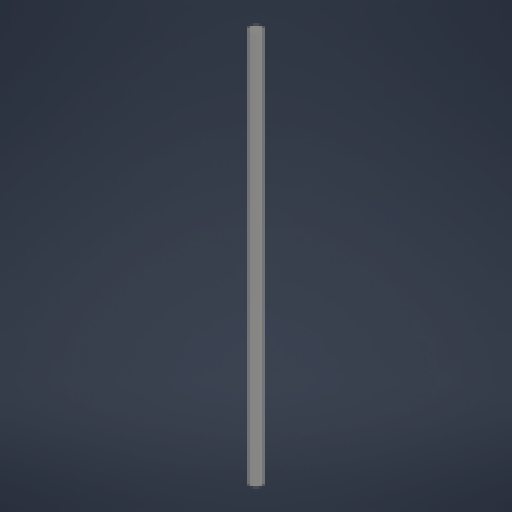
# Autodesk Inventor part: bar
Saved by Autodesk Inventor 2023 (Build 270158030, 158C)
## iProperties
Created: 2022-04-23
Part Number: bar
Material: Stainless Steel
Document SubType Name: Modeling
Designer: Norbert Ligas
Density: 8 g/cm^3
Appearance: Semi-Polished
Mass: 114.605 g
Surface Area: 72.6336 cm^2
Volume: 14.3257 cm^3
bar_length: 265,000
bar_diameter: 8,000 mm
Author: Norbert Ligas
Autodesk Inventor part; units mm, degrees
ref_plane "YZ Plane" through (0, 0, 0) normal (1, 0, 0) x (0, 1, 0)
ref_plane "XZ Plane" through (0, 0, 0) normal (0, 1, 0) x (-1, 0, 0)
ref_plane "XY Plane" through (0, 0, 0) normal (0, 0, 1) x (1, 0, 0)
sketch "Sketch1" plane through (0, 0, 0) normal (0, 1, 0) x (-1, 0, 0)
  circle A0 centre (0, 0) radius 4
  dimension "d0" = 8
  constraints: 1 centre point, 1 coincident
  measures "d0" diameter of A0
extrude "Extrusion1" add sketch "Sketch1" along normal blind 265
equation "\"d0\" = bar_diameter"
equation "\"d1\" = bar_length"
equation "\"bar_length\" = -hinge_insertion + pipe_length + connection_length"
equation "\"bar_diameter\" = 8"
equation "\"hinge_insertion\" = 15"
equation "\"pipe_length\" = 260"
equation "\"connection_length\" = 20"
body "Solid1"
